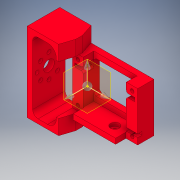
# Autodesk Inventor part: EDMO1-1_Body
Saved by Autodesk Inventor 2019 (Build 230136000, 136)
## iProperties
Created: 2016-10-24
Part Number: EDMO1-1_Body
Material: PLA
Document SubType Name: Modeling
Designer: Lucas
Density: 1.29985 g/cm^3
Appearance: Generic
Mass: 64.7443 g
Surface Area: 221.081 cm^2
Volume: 49.8091 cm^3
Author: Lucas
Autodesk Inventor part; units mm, degrees
ref_plane "YZ Plane" through (0, 0, 0) normal (1, 0, 0) x (0, 1, 0)
ref_plane "XZ Plane" through (0, 0, 0) normal (0, 1, 0) x (-1, 0, 0)
sketch "Sketch2" plane through (0, 0, 0) normal (0, 0, 1) x (1, 0, 0)
  line L0 (0, 0) -> (60, 0)
  line L1 (60, 0) -> (60, 45)
  line L2 (60, 45) -> (0, 45)
  line L3 (0, 45) -> (0, 0)
  dimension "d0" = 60
  dimension "d1" = 45
  constraints: 8 end point, 2 parallel, 1 horizontal, 1 perpendicular
  measures "d0" distance of L2.end L1.end
  measures "d1" distance of L1.end L0.end
extrude "Body_body" add sketch "Sketch2" along normal blind 15
sketch "Sketch4" plane through (0, 0, 15) normal (0, 0, 1) x (1, 0, 0)
  line L0 (60, 45) -> (0, 45) projected
  line L1 (0, 45) -> (0, 0) projected
  line L2 (2.05, 33.35) -> (9.75, 33.35)
  line L3 (9.75, 33.35) -> (9.75, 4.9)
  line L4 (9.75, 4.9) -> (49.55, 4.9)
  line L5 (49.55, 4.9) -> (49.55, 33.35)
  line L6 (49.55, 33.35) -> (57.25, 33.35)
  line L7 (60, 0) -> (60, 45) projected
  line L8 (0, 0) -> (60, 0) projected
  line L9 (2.05, 33.35) -> (2.05, 36.65)
  line L10 (2.05, 36.65) -> (9.75, 36.65)
  line L11 (9.75, 36.65) -> (9.75, 45)
  line L12 (57.25, 36.65) -> (57.25, 33.35)
  line L13 (57.25, 36.65) -> (49.55, 36.65)
  line L14 (49.55, 36.65) -> (49.55, 45)
  line L15 (9.75, 45) -> (49.55, 45)
  line L16 (30, 36.5125) -> (30, -47.625) construction
  line L17 (-8.6434, 35) -> (87.0327, 35) construction
  point P0 (45, 45)
  dimension "d6" = 7.7
  dimension "d8" = 39.8
  dimension "d11" = 4.9
  dimension "d14" = 3.3
  dimension "d15" = 3.3
  dimension "d22" = 60
  dimension "d23" = 30
  dimension "d25" = 20.25
  dimension "d28" = 7.7
  dimension "d213" = 40.1
  dimension "d246" = 1.65
  dimension "d247" = 31.75
  dimension "d248" = 28.45
  dimension "d250" = 10
  constraints: 28 end point, 5 collinear, 5 horizontal, 5 perpendicular, 3 point on line, 2 vertical, 1 other
  measures "d6" distance of L2.start L2.end
  measures "d8" distance of L3.end L4.end
  measures "d11" distance between parallel lines of L8 L4
  measures "d14" distance of L2.start L9.end
  measures "d15" distance of L12.start L6.end
  measures "d22" distance between parallel lines of L7 L1
  measures "d23" distance between parallel lines of L16 L1
  measures "d25" distance between parallel lines of L16 L11
  measures "d28" distance of L12.start L13.end
  measures "d213" distance between parallel lines of L4 L15
  measures "d246" distance between parallel lines of L17 L2
  measures "d247" distance between parallel lines of L10 L4
  measures "d248" distance between parallel lines of L2 L4
  measures "d250" distance between parallel lines of L0 L17
extrude "Servo_Intake" cut sketch "Sketch4" against normal blind 9.85 contours L14 L13 L12 L6 L5 L4 L3 L2 L9 L10 L11 L0
sketch "Sketch5" plane through (0, 0, 15) normal (0, 0, 1) x (1, 0, 0)
  line L0 (60, 8.9) -> (60, 5.9)
  line L1 (-29.647, 7.4) -> (54.8226, 7.4) construction
  line L2 (0, 0) -> (60, 0) projected
  line L3 (49.55, 4.9) -> (9.75, 4.9) projected
  line L4 (60, 5.9) -> (49.55, 5.9)
  line L5 (49.55, 5.9) -> (49.55, 8.9)
  line L6 (49.55, 33.35) -> (49.55, 4.9) projected
  line L7 (60, 8.9) -> (49.55, 8.9)
  line L8 (60, 0) -> (60, 45) projected
  dimension "d171" = 3
  dimension "d271" = 7.4
  constraints: 10 end point, 1 collinear, 1 horizontal, 1 perpendicular, 1 point on line, 1 other
  measures "d171" distance between parallel lines of L7 L4
  measures "d271" distance between parallel lines of L1 L2
extrude "Cable_Opening" cut sketch "Sketch5" against normal blind 4
sketch "Sketch6" plane through (0, 0, 15) normal (0, 0, 1) x (1, 0, 0)
  circle A0 centre (5, 40.75) radius 1.7
  circle A1 centre (55, 40.75) radius 1.7
  circle A2 centre (55, 4.25) radius 1.7
  circle A3 centre (5, 4.25) radius 1.7
  line L0 (30, 47.1) -> (30, -0.525) construction
  line L1 (-16.6375, 22.5) -> (70.675, 22.5) construction
  line L2 (60, 8.9) -> (60, 45) projected
  line L3 (0, 45) -> (0, 0) projected
  line L4 (9.75, 45) -> (0, 45) projected
  line L5 (0, 0) -> (60, 0) projected
  point P0 (42, 12.35)
  point P1 (60, 45)
  point P2 (0, 12.35)
  dimension "d29" = 3.4
  dimension "d30" = 3.4
  dimension "d31" = 3.4
  dimension "d32" = 3.4
  dimension "d33" = 60
  dimension "d34" = 30
  dimension "d35" = 45
  dimension "d36" = 22.5
  dimension "d37" = 50
  dimension "d38" = 25
  dimension "d39" = 36.5
  dimension "d40" = 18.25
  constraints: 4 centre point, 4 end point, 2 horizontal alignment, 2 vertical alignment, 1 horizontal, 1 other
  measures "d29" diameter of A0
  measures "d30" diameter of A1
  measures "d31" diameter of A2
  measures "d32" diameter of A3
  measures "d34" distance between parallel lines of L0 L3
  measures "d35" distance between parallel lines of L4 L5
  measures "d36" distance between parallel lines of L4 L1
  measures "d37" distance of A1.centre A0.centre
  measures "d38" distance from line of L0 A0.centre
  measures "d39" distance of A3.centre A0.centre
  measures "d40" distance from line of L1 A2.centre
extrude "Holes_Cover_Screws" cut sketch "Sketch6" against normal up to surface (15 mm away)
sketch "Sketch10" plane through (0, 0, 15) normal (0, 0, 1) x (1, 0, 0)
  line L0 (50.25, 4.9) -> (9.75, 4.9)
  line L1 (50.25, 0) -> (9.75, 0)
  line L2 (9.75, 4.9) -> (9.75, 33.35) projected
  line L3 (49.55, 33.35) -> (49.55, 4.9) projected
  line L4 (0, 0) -> (60, 0) projected
  line L5 (9.75, 0) -> (9.75, 4.9)
  line L6 (50.25, 0) -> (50.25, 4.9)
  line L7 (49.55, 4.9) -> (9.75, 4.9) projected
  line L8 (30, 50.585) -> (30, -19.2942) construction
  line L9 (60, 8.9) -> (60, 45) projected
  line L10 (0, 45) -> (0, 0) projected
  dimension "d214" = 60
  dimension "d215" = 30
  constraints: 10 end point, 3 collinear, 2 vertical, 1 parallel, 1 other
  measures "d214" distance between parallel lines of L9 L10
  measures "d215" distance between parallel lines of L8 L10
extrude "Socket" add sketch "Sketch10" along normal blind 10
sketch "Sketch11" plane through (9.75, 4.9, 5.15) normal (0, 1, 0) x (1, 0, 0)
  circle A0 centre (29.3, -9.9) radius 1.55
  line L0 (50.25, 5.15) -> (50.25, -9.85) projected
  line L1 (39.8, 0) -> (0, 0) projected
  point P0 (-9.75, 5.15)
  dimension "d65" = 3.1
  dimension "d217" = 9.9
  dimension "d256" = 20.95
  constraints: 1 centre point
  measures "d65" diameter of A0
  measures "d217" distance from line of A0.centre L1
  measures "d256" distance from line of L0 A0.centre
extrude "Hole_Shaft" cut sketch "Sketch11" against normal up to surface (4.9 mm away)
sketch "Sketch12" plane through (9.75, 4.9, 5.15) normal (0, 1, 0) x (1, 0, 0)
  circle A0 centre (29.3, -9.9) radius 4
  circle A1 centre (29.3, -9.9) radius 1.55 projected
  point P0 (-9.75, 5.15)
  dimension "d73" = 8
  constraints: 1 centre point, 1 concentric
  measures "d73" diameter of A0
extrude "Pocket_Shaft" cut sketch "Sketch12" against normal blind 3.2
sketch "Sketch15" plane through (0, 0, 15) normal (0, 0, 1) x (1, 0, 0)
  line L0 (9.75, 45) -> (0, 45) projected
  line L1 (0, 0) -> (9.75, 0) projected
  line L2 (60, 45) -> (49.55, 45) projected
  line L3 (0, 0) -> (60, 0) projected
  line L4 (60, 45) -> (0, 45) projected
  line L5 (0, 45) -> (0, 55)
  line L6 (0, 55) -> (-21.8, 55)
  line L7 (0, 45) -> (6, 45)
  line L8 (6, 45) -> (6, 59)
  line L9 (6, 59) -> (-26.8, 59)
  line L10 (0, 0) -> (0, -10)
  line L11 (0, -10) -> (-21.8, -10)
  line L12 (-21.8, -10) -> (-21.8, 55)
  line L13 (0, 0) -> (6, 0)
  line L14 (6, 0) -> (6, -14)
  line L15 (6, -14) -> (-26.8, -14)
  line L16 (-26.8, -14) -> (-26.8, 59)
  line L17 (0, 45) -> (0, 0) projected
  point P0 (0, 5.5)
  point P1 (60, 0)
  point P2 (13.5, 8)
  point P3 (36.5, 8)
  dimension "d111" = 10
  dimension "d113" = 6
  dimension "d114" = 14
  dimension "d116" = 10
  dimension "d117" = 21.8
  dimension "d118" = 6
  dimension "d119" = 14
  dimension "d120" = 32.8
  dimension "d161" = 4
  dimension "d175" = 32.8
  dimension "d191" = 5
  constraints: 24 end point, 7 perpendicular, 2 parallel, 1 collinear, 1 point on line, 1 vertical, 3 other
  measures "d111" distance of L0.end L5.end
  measures "d113" distance of L0.end L7.end
  measures "d114" distance of L7.end L8.end
  measures "d116" distance of L10.start L10.end
  measures "d117" distance of L10.end L11.end
  measures "d118" distance of L10.start L13.end
  measures "d119" distance of L13.end L14.end
  measures "d120" distance of L14.end L15.end
  measures "d161" distance between parallel lines of L15 L11
  measures "d175" distance of L8.end L9.end
  measures "d191" distance between parallel lines of L16 L12
extrude "Connector" add sketch "Sketch15" along normal mid plane 30 contours L0 L5 L6 L12 L11 L10 L1 L14 L15 L16 L9 L8
sketch "Sketch17" plane through (-21.8, -10, 30) normal (1, 0, 0) x (0, 0, -1)
  circle A0 centre (15, 32.5) radius 11 construction
  line L0 (30, 65) -> (0, 65) projected
  line L1 (30, 0) -> (0, 0) projected
  line L2 (0, 0) -> (0, 65) projected
  line L3 (30, 65) -> (30, 0) projected
  line L4 (15, 19.142) -> (15, 44.542) construction
  line L5 (1.1452, 32.5) -> (27.1241, 32.5) construction
  line L6 (4.9901, 22.4901) -> (35.9566, 53.4566) construction
  line L7 (5.2574, 42.2426) -> (22.7782, 24.7218) construction
  circle A1 centre (7.2218, 24.7218) radius 1.85
  circle A2 centre (4, 32.5) radius 1.85
  circle A3 centre (7.2218, 40.2782) radius 1.85
  circle A4 centre (15, 43.5) radius 1.85
  circle A5 centre (15, 21.5) radius 1.85
  circle A6 centre (22.7782, 24.7218) radius 1.85
  circle A7 centre (26, 32.5) radius 1.85
  circle A8 centre (22.7782, 40.2782) radius 1.85
  point P0 (30, 10)
  dimension "d121" = 22
  dimension "d122" = 65
  dimension "d123" = 32.5
  dimension "d124" = 30
  dimension "d125" = 15
  dimension "d126" = 3.7
  dimension "d127" = 3.7
  dimension "d128" = 3.7
  dimension "d129" = 3.7
  dimension "d130" = 3.7
  dimension "d131" = 3.7
  dimension "d132" = 3.7
  dimension "d133" = 3.7
  dimension "d134" = 45
  dimension "d135" = 45
  constraints: 11 point on line, 8 centre point, 8 end point, 1 coincident, 1 horizontal, 1 vertical, 10 other
  measures "d122" distance between parallel lines of L0 L1
  measures "d123" distance from line of point (15, 32.5) L1
  measures "d124" distance between parallel lines of L2 L3
  measures "d125" distance from line of L2 point (15, 32.5)
  measures "d126" diameter of A1
  measures "d127" diameter of A2
  measures "d128" diameter of A3
  measures "d129" diameter of A4
  measures "d130" diameter of A5
  measures "d131" diameter of A6
  measures "d132" diameter of A7
  measures "d133" diameter of A8
  measures "d134" angle of L6 L4
  measures "d135" angle of L4 L7
extrude "Connector_Holes" cut sketch "Sketch17" against normal up to surface (5 mm away) contours A1 | A2 | A3 | A4 | A5 | A6 | A7 | A8
sketch "Sketch19" plane through (-21.8, -10, 30) normal (1, 0, 0) x (0, 0, -1)
  circle A0 centre (15, 32.5) radius 5
  line L0 (30, 0) -> (0, 0) projected
  line L1 (30, 65) -> (0, 65) projected
  line L2 (30, 65) -> (30, 0) projected
  line L3 (0, 0) -> (0, 65) projected
  point P0 (30, 10)
  dimension "d140" = 10
  dimension "d141" = 65
  dimension "d142" = 32.5
  dimension "d143" = 30
  dimension "d144" = 15
  constraints: 1 centre point
  measures "d140" diameter of A0
  measures "d141" distance between parallel lines of L0 L1
  measures "d142" distance from line of L1 A0.centre
  measures "d143" distance between parallel lines of L2 L3
  measures "d144" distance from line of L3 A0.centre
extrude "Connector_Center_Hole" cut sketch "Sketch19" against normal up to surface (5 mm away) contours A0
sketch "Sketch23" plane through (0, 0, 30) normal (0, 0, 1) x (1, 0, 0)
  line L0 (0, 45) -> (6, 45) projected
  line L1 (6, 45) -> (0, 45)
  line L2 (0, 45) -> (0, 45.25)
  line L3 (0, 45.25) -> (6, 45.25)
  line L4 (6, 45.25) -> (6, 45)
  line L5 (6, -14) -> (6, 0) projected
  line L6 (0, 0) -> (6, 0)
  line L7 (6, 0) -> (6, -0.25)
  line L8 (6, -0.25) -> (0, -0.25)
  line L9 (0, -0.25) -> (0, 0)
  point P0 (6, -8)
  dimension "d162" = 0.25
  dimension "d163" = 0.25
  constraints: 16 end point, 4 parallel, 2 horizontal, 2 perpendicular, 1 point on line
  measures "d162" distance between parallel lines of L0 L3
  measures "d163" distance between parallel lines of L6 L8
extrude "Material_Reduction_CoverFit01" cut sketch "Sketch23" against normal up to surface (15 mm away)
fillet "Fillet4" radius 8 2 edges at (0, 55, 15) (0, -10, 15)
chamfer "Chamfer1" distance 12 angle 18 1 edges at (6, -7.125, 30) measured on face at (6, -9.4167, 15)
chamfer "Chamfer2" distance 12 angle 18 1 edges at (6, -7, 0) measured on face at (6, -9.4167, 11)
chamfer "Chamfer3" distance 12 angle 18 1 edges at (6, 52.125, 30) measured on face at (6, 54.4167, 15)
chamfer "Chamfer4" distance 12 angle 18 1 edges at (6, 52, 0) measured on face at (6, 54.4167, 11)
fillet "Fillet5" radius 5 2 edges at (-21.8, -10, 15) (-21.8, 55, 15)
sketch "Sketch31" plane through (0, 0, 25) normal (0, 0, 1) x (1, 0, 0)
  line L0 (9.75, 0) -> (9.75, 4.9) projected
  line L1 (9.75, 4.9) -> (50.25, 4.9)
  line L2 (50.25, 4.9) -> (50.25, 0)
  line L3 (50.25, 0) -> (9.75, 0)
  line L4 (9.75, 0) -> (9.75, 4.9)
  line L5 (9.75, 0) -> (50.25, 0) projected
  line L6 (50.25, 0) -> (50.25, 4.9) projected
  point P0 (0, 0)
  constraints: 8 end point, 2 collinear, 2 parallel, 1 horizontal, 1 perpendicular
extrude "Material_Reduction_CoverFit02" cut sketch "Sketch31" against normal blind 0.4
sketch "Sketch33" plane through (0, 0, 5.15) normal (0, 0, 1) x (1, 0, 0)
  line L0 (9.3181, 40) -> (49.3181, 40)
  line L1 (49.55, 40) -> (9.75, 40)
  line L2 (9.75, 40) -> (9.75, 9.9)
  line L3 (9.75, 9.9) -> (49.55, 9.9)
  line L4 (49.55, 9.9) -> (49.55, 40)
  line L5 (49.55, 4.9) -> (9.75, 4.9) projected
  line L6 (49.55, 33.35) -> (49.55, 4.9) projected
  line L7 (9.75, 4.9) -> (9.75, 33.35) projected
  line L8 (9.75, 45) -> (49.55, 45) projected
  point P0 (0, 0)
  dimension "d258" = 5
  dimension "d259" = 5
  constraints: 10 end point, 2 collinear, 2 parallel, 1 horizontal, 1 perpendicular, 1 point on line
  measures "d258" distance between parallel lines of L5 L3
  measures "d259" distance between parallel lines of L0 L8
extrude "Cooling_Opening" cut sketch "Sketch33" against normal up to surface (5.15 mm away) contours L0 L1 L4 L3 L2
chamfer "Chamfer5" distance 2 angle 45 4 edges at (9.75, 40, 2.575) (49.55, 40, 2.575) (9.75, 9.9, 2.575) (49.55, 9.9, 2.575)
ref_plane "Work Plane2" through (60, 22.5, 0) normal (0, -1, 0) x (1, 0, 0)
sketch "Sketch34" plane through (0, 0, 24.6) normal (0, 0, 1) x (1, 0, 0)
  line L0 (9.75, 0) -> (9.75, 4.9) projected
  line L1 (2.101, 0) -> (60, 0) projected
  line L2 (9.75, 4.9) -> (10.25, 4.9)
  line L3 (10.25, 4.9) -> (10.25, 0)
  line L4 (10.25, 0) -> (9.75, 0)
  line L5 (9.75, 0) -> (9.75, 4.9)
  line L6 (9.75, 4.9) -> (50.25, 4.9) projected
  line L7 (50.25, 0) -> (49.25, 0)
  line L8 (49.25, 0) -> (49.25, 4.9)
  line L9 (49.25, 4.9) -> (50.25, 4.9)
  line L10 (50.25, 4.9) -> (50.25, 0)
  line L11 (50.25, 4.9) -> (50.25, 0) projected
  point P0 (0, 0)
  dimension "d265" = 0.5
  dimension "d266" = 1
  constraints: 16 end point, 4 parallel, 3 point on line, 2 horizontal, 2 perpendicular, 1 collinear
  measures "d265" distance between parallel lines of L0 L3
  measures "d266" distance between parallel lines of L10 L8
extrude "Material_Reduction_CoverFit03" cut sketch "Sketch34" against normal up to surface (9.6 mm away) contours L0 L2 L3 L1 | L8 L6 L10 L1
fillet "Fillet7" radius 2 4 edges at (9.75, 33.35, 10.075) (9.75, 36.65, 10.075) (49.55, 33.35, 10.075) (49.55, 36.65, 10.075)
sketch "Sketch35" plane through (0, 0, 0) normal (0, 0, -1) x (-1, 0, 0)
  circle A0 centre (-5, 4.25) radius 1.7 projected
  line L0 (-7.71, 5.8146) -> (-5, 7.3792)
  line L1 (-5, 7.3792) -> (-2.29, 5.8146)
  line L2 (-2.29, 5.8146) -> (-2.29, 2.6854)
  line L3 (-2.29, 2.6854) -> (-5, 1.1208)
  line L4 (-5, 1.1208) -> (-7.71, 2.6854)
  line L5 (-7.71, 2.6854) -> (-7.71, 5.8146)
  line L6 (-2.101, 0) -> (-60, 0) projected
  line L7 (0, -2) -> (0, 47) projected
  circle A1 centre (-55, 4.25) radius 1.7 projected
  line L8 (-57.71, 2.6854) -> (-57.71, 5.8146)
  line L9 (-57.71, 5.8146) -> (-55, 7.3792)
  line L10 (-55, 7.3792) -> (-52.29, 5.8146)
  line L11 (-52.29, 5.8146) -> (-52.29, 2.6854)
  line L12 (-52.29, 2.6854) -> (-55, 1.1208)
  line L13 (-55, 1.1208) -> (-57.71, 2.6854)
  circle A2 centre (-55, 40.75) radius 1.7 projected
  line L14 (-57.71, 39.1854) -> (-57.71, 42.3146)
  line L15 (-57.71, 42.3146) -> (-55, 43.8792)
  line L16 (-55, 43.8792) -> (-52.29, 42.3146)
  line L17 (-52.29, 42.3146) -> (-52.29, 39.1854)
  line L18 (-52.29, 39.1854) -> (-55, 37.6208)
  line L19 (-55, 37.6208) -> (-57.71, 39.1854)
  circle A3 centre (-5, 40.75) radius 1.7 projected
  line L20 (-7.71, 39.1854) -> (-7.71, 42.3146)
  line L21 (-7.71, 42.3146) -> (-5, 43.8792)
  line L22 (-5, 43.8792) -> (-2.29, 42.3146)
  line L23 (-2.29, 42.3146) -> (-2.29, 39.1854)
  line L24 (-2.29, 39.1854) -> (-5, 37.6208)
  line L25 (-5, 37.6208) -> (-7.71, 39.1854)
  point P0 (0, 0)
  dimension "d270" = 5.42
  dimension "d275" = 5.42
  dimension "d276" = 5.42
  dimension "d277" = 5.42
  constraints: 48 end point, 4 coincident, 4 parallel, 52 other
  measures "d270" distance between parallel lines of L0 L3
  measures "d275" distance between parallel lines of L9 L12
  measures "d276" distance between parallel lines of L21 L24
  measures "d277" distance between parallel lines of L15 L18
extrude "Pockets_Nuts" cut sketch "Sketch35" against normal blind 7 contours A0 | L0 L1 L2 L3 L4 L5 | A1 | L8 L9 L10 L11 L12 L13 | A2 | L14 L15 L16 L17 L18 L19 | A3 | L20 L21 L22 L23 L24 L25
chamfer "Chamfer6" distance 1 angle 45 24 edges at (56.355, 6.5969, 0) (57.71, 4.25, 0) (56.355, 1.9031, 0) (53.645, 1.9031, 0) (52.29, 4.25, 0) (53.645, 6.5969, 0) (56.355, 43.0969, 0) (57.71, 40.75, 0) (56.355, 38.4031, 0) (53.645, 38.4031, 0) (52.29, 40.75, 0) (53.645, 43.0969, 0) (6.355, 6.5969, 0) (7.71, 4.25, 0) (6.355, 1.9031, 0) (3.645, 1.9031, 0) (2.29, 4.25, 0) (3.645, 6.5969, 0) (7.71, 40.75, 0) (6.355, 43.0969, 0) (3.645, 43.0969, 0) (2.29, 40.75, 0) (3.645, 38.4031, 0) (6.355, 38.4031, 0)
equation "\"d15\" = d14"
equation "\"d23\" = 0.5 * d22"
equation "\"d25\" = 0.5 * d24"
equation "\"d28\" = d6"
equation "\"d34\" = 0.5 * d33"
equation "\"d36\" = 0.5 * d35"
equation "\"d38\" = 0.5 * d37"
equation "\"d40\" = 0.5 * d39"
equation "\"d123\" = 0.5 * d122"
equation "\"d125\" = 0.5 * d124"
equation "\"d142\" = 0.5 * d141"
equation "\"d144\" = 0.5 * d143"
equation "\"d24\" = 40.5"
body "Solid1"
